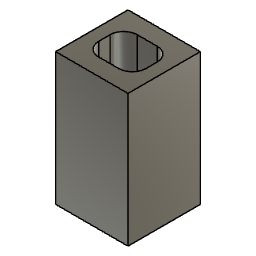
motorPiece v2 (Autodesk Fusion 360 design; units mm, degrees)
Autodesk Fusion 360 part; units mm, degrees
sketch "Sketch4" plane through (0, 0, 0) normal (0, 0, 1) x (1, 0, 0)
  line L0 (-82, 90) -> (-90, 90)
  line L1 (-90, 90) -> (-90, 82)
  line L2 (-90, 82) -> (-82, 82)
  line L3 (-82, 82) -> (-82, 90)
  dimension "d5" = 8
  dimension "d6" = 8
  constraint horizontal L0
  constraint perpendicular L0 L1
  constraint parallel L0 L2
  constraint parallel L1 L3
  measures "d5" distance of L1 L3
  measures "d6" distance of L0 L2
extrude "Extrude2" add sketch "Sketch4" along normal blind 14.625
sketch "Sketch5" plane through (0, 0, 14.625) normal (0, 0, 1) x (-1, 0, 0)
  line L0 (82, -82) -> (82, -90)
  line L1 (82, -90) -> (90, -90)
  line L2 (90, -90) -> (90, -82)
  line L3 (90, -82) -> (82, -82)
move_body "Move1" bodies 1 to x (1, 0, 0) y (0, 1, 0) z (0, 0, 1) at (86, -86, 0)
sketch "Sketch7" plane through (0, 0, 14.625) normal (0, 0, 1) x (-1, 0, 0)
  line L0 (-4, 4) -> (-4, -4)
  line L1 (-4, -4) -> (4, -4)
  line L2 (4, -4) -> (4, 4)
  line L3 (4, 4) -> (-4, 4)
  line L4 (1.11, -2.13) -> (-1.11, -2.13)
  line L5 (-2.61, -0.63) -> (-2.61, 0.63)
  line L6 (-1.11, 2.13) -> (1.11, 2.13)
  line L7 (2.61, 0.63) -> (2.61, -0.63)
  circle A0 centre (0, 0) radius 0.98
  arc A1 (1.11, -2.13) -> (2.61, -0.63) centre (1.11, -0.63) ccw
  arc A2 (-2.61, -0.63) -> (-1.11, -2.13) centre (-1.11, -0.63) ccw
  arc A3 (-1.11, 2.13) -> (-2.61, 0.63) centre (-1.11, 0.63) ccw
  arc A4 (2.61, 0.63) -> (1.11, 2.13) centre (1.11, 0.63) ccw
  point P0 (-2.61, -2.13)
  point P1 (-2.61, 2.13)
  point P2 (2.61, 2.13)
  dimension "d7" = 5.22
  dimension "d8" = 4.26
  dimension "d9" = 1.96
  dimension "d10" = 1.5
  constraint horizontal L4
  constraint perpendicular L4 L5
  constraint parallel L4 L6
  constraint parallel L5 L7
  constraint coincident A0.centre origin
  constraint tangent L4 A1
  constraint tangent L7 A1
  constraint coincident P0 L4
  constraint coincident P0 L5
  constraint tangent L4 A2
  constraint tangent L5 A2
  constraint equal A1 A2
  constraint coincident P1 L5
  constraint coincident P1 L6
  constraint tangent L5 A3
  constraint tangent L6 A3
  constraint equal A1 A3
  constraint coincident P2 L6
  constraint coincident P2 L7
  constraint tangent L6 A4
  constraint tangent L7 A4
  constraint equal A1 A4
  measures "d7" distance of P1 P2
  measures "d8" distance of P0 P1
  measures "d9" diameter of A0
  measures "d10" radius of A1
extrude "Extrude3" cut sketch "Sketch7" along normal blind 0 and the other way blind 7.3125 contours L4 L5 L6 L7 A1 A2 A3 A4 | A0
sketch "Sketch8" plane through (0, 0, 0) normal (0, 0, -1) x (1, 0, 0)
  line L0 (4, -4) -> (4, 4)
  line L1 (4, 4) -> (-4, 4)
  line L2 (-4, 4) -> (-4, -4)
  line L3 (-4, -4) -> (4, -4)
  line L4 (-1.585, 1.585) -> (1.585, 1.585)
  line L5 (1.585, 1.585) -> (1.585, -1.585)
  line L6 (1.585, -1.585) -> (-1.585, -1.585)
  line L7 (-1.585, -1.585) -> (-1.585, 1.585)
  line L8 (-1.585, 1.585) -> (1.585, -1.585) construction
  line L9 (1.585, 1.585) -> (-1.585, -1.585) construction
  dimension "d15" = 3.17
  constraint horizontal L4
  constraint perpendicular L4 L5
  constraint parallel L4 L6
  constraint parallel L5 L7
  constraint coincident L8 origin
  constraint coincident L9 origin
  measures "d15" distance of L4 L6
extrude "Extrude4" cut sketch "Sketch8" along normal blind 0 and the other way blind 5.6562 contours L4 L5 L6 L7
